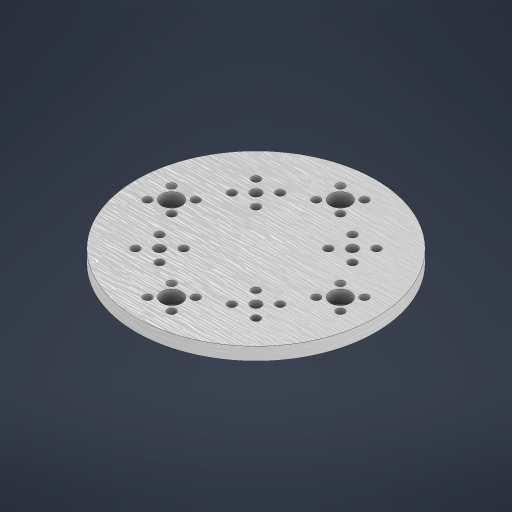
# Autodesk Inventor part: TurnTable
Saved by Autodesk Inventor 2024 (Build 280153000, 153)
## iProperties
Created: 2023-10-18
Part Number: TurnTable
Material: Generic
Document SubType Name: Modeling
Designer: avsar
Density: 1 g/cm^3
Appearance: Polished Brushed
Author: avsar
Autodesk Inventor part; units mm, degrees
ref_plane "YZ Plane" through (0, 0, 0) normal (1, 0, 0) x (0, 1, 0)
ref_plane "XZ Plane" through (0, 0, 0) normal (0, 1, 0) x (-1, 0, 0)
ref_plane "XY Plane" through (0, 0, 0) normal (0, 0, 1) x (1, 0, 0)
sketch "Sketch1" plane through (0, 0, 0) normal (0, 1, 0) x (-1, 0, 0)
  circle A0 centre (0, 0) radius 59.5
  dimension "d0" = 119
  constraints: 1 centre point, 1 coincident
  measures "d0" diameter of A0
extrude "Extrusion1" add sketch "Sketch1" along normal mid plane 6.35
sketch "Sketch5" plane through (0, 3.175, 0) normal (0, 1, 0) x (1, 0, 0)
  circle A0 centre (-42, 0) radius 5
  circle A1 centre (-36, 6) radius 2
  circle A2 centre (-48, 6) radius 2
  circle A3 centre (-48, -6) radius 2
  circle A4 centre (-36, -6) radius 2
  circle A5 centre (0, -42) radius 5
  circle A6 centre (-6, -36) radius 2
  circle A7 centre (-6, -48) radius 2
  circle A8 centre (6, -48) radius 2
  circle A9 centre (6, -36) radius 2
  circle A10 centre (42, 0) radius 5
  circle A11 centre (36, -6) radius 2
  circle A12 centre (48, -6) radius 2
  circle A13 centre (48, 6) radius 2
  circle A14 centre (36, 6) radius 2
  circle A15 centre (0, 42) radius 5
  circle A16 centre (6, 36) radius 2
  circle A17 centre (6, 48) radius 2
  circle A18 centre (-6, 48) radius 2
  circle A19 centre (-6, 36) radius 2
  point P0 (0, 0)
  dimension "d37" = 10
  dimension "d38" = 42
  dimension "d39" = 4
  dimension "d40" = 6
  dimension "d41" = 6
  dimension "d44" = 360
  dimension "d48" = 360
  constraints: 20 centre point, 1 horizontal alignment, 50 other
  measures "d37" diameter of A0
  measures "d38" distance of point (0, 0) A0.centre
  measures "d39" diameter of A1
  measures "d40" horizontal distance of A0.centre A1.centre
  measures "d41" horizontal distance of A0.centre A1.centre
extrude "Extrusion4" cut sketch "Sketch5" against normal through all
sketch "Sketch8" plane through (0, 3.175, 0) normal (0, 1, 0) x (1, 0, 0)
  circle A0 centre (-24, -24) radius 2.5
  circle A1 centre (-30, -18) radius 2
  circle A2 centre (-30, -30) radius 2
  circle A3 centre (-18, -30) radius 2
  circle A4 centre (-18, -18) radius 2
  circle A5 centre (24, -24) radius 2.5
  circle A6 centre (18, -30) radius 2
  circle A7 centre (30, -30) radius 2
  circle A8 centre (30, -18) radius 2
  circle A9 centre (18, -18) radius 2
  circle A10 centre (24, 24) radius 2.5
  circle A11 centre (30, 18) radius 2
  circle A12 centre (30, 30) radius 2
  circle A13 centre (18, 30) radius 2
  circle A14 centre (18, 18) radius 2
  circle A15 centre (-24, 24) radius 2.5
  circle A16 centre (-18, 30) radius 2
  circle A17 centre (-30, 30) radius 2
  circle A18 centre (-30, 18) radius 2
  circle A19 centre (-18, 18) radius 2
  point P0 (0, 0)
  dimension "d70" = 5
  dimension "d71" = 24
  dimension "d72" = 24
  dimension "d73" = 4
  dimension "d74" = 6
  dimension "d75" = 6
  dimension "d78" = 360
  dimension "d88" = 360
  constraints: 20 centre point, 50 other
  measures "d70" diameter of A0
  measures "d71" horizontal distance of point (0, 0) A0.centre
  measures "d72" horizontal distance of point (0, 0) A0.centre
  measures "d73" diameter of A1
  measures "d74" horizontal distance of A1.centre A0.centre
  measures "d75" horizontal distance of A0.centre A1.centre
extrude "Extrusion6" cut sketch "Sketch8" against normal through all
body "Solid1"
